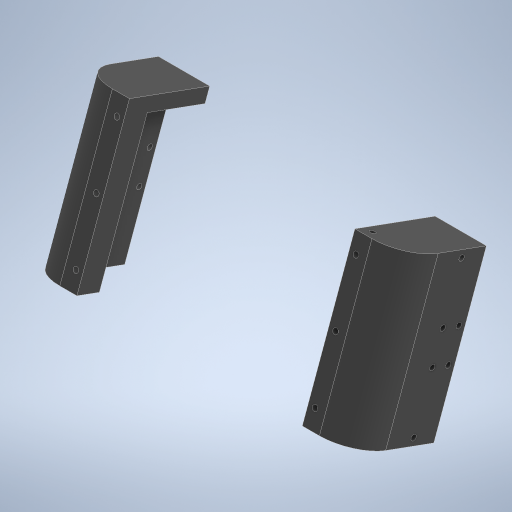
# Autodesk Inventor part: chest_cover_side
Saved by Autodesk Inventor 2024.1 (Build 281209000, 209)
## iProperties
Created: 2024-02-14
Part Number: chest_cover_side
Material: 一般
Document SubType Name: Modeling
Designer: hibik
Density: 1 g/cm^3
Appearance: 既定
Author: hibik
Autodesk Inventor part; units mm, degrees
ref_plane "YZ Plane" through (0, 0, 0) normal (1, 0, 0) x (0, 1, 0)
ref_plane "XZ Plane" through (0, 0, 0) normal (0, 1, 0) x (-1, 0, 0)
ref_plane "XY Plane" through (0, 0, 0) normal (0, 0, 1) x (1, 0, 0)
sketch "スケッチ1" plane through (0, 0, 0) normal (1, 0, 0) x (0, 1, 0)
  line L0 (0, 0) -> (33, 0)
  line L1 (33, 0) -> (3.8603, 10.606)
  line L2 (3.8603, 10.606) -> (0, 0)
  line L3 (33, 0) -> (3.8603, 10.606)
  line L4 (3.8603, 10.606) -> (5.2283, 14.3648)
  line L5 (5.2283, 14.3648) -> (34.3681, 3.7588)
  line L6 (34.3681, 3.7588) -> (33, 0)
  line L7 (5.2283, 14.3648) -> (0, 12.011)
  line L8 (0, 12.011) -> (3.8603, 10.606)
  line L9 (0, 0) -> (0, 12.011)
  circle A0 centre (2, 10.7181) radius 0.8
  line L10 (34.3681, 3.7588) -> (42.9186, 27.2511)
  line L11 (42.9186, 27.2511) -> (8.15, 39.9058)
  line L12 (8.15, 39.9058) -> (-0.4005, 16.4135)
  line L13 (-0.4005, 16.4135) -> (34.3681, 3.7588)
  line L14 (-0.4005, 16.4135) -> (8.15, 39.9058)
  line L15 (8.15, 39.9058) -> (50.4361, 24.5149)
  line L16 (50.4361, 24.5149) -> (41.8856, 1.0226)
  line L17 (41.8856, 1.0226) -> (-0.4005, 16.4135)
  line L18 (8.15, 39.9058) -> (-1.9502, 12.1558)
  line L19 (-1.9502, 12.1558) -> (2, 10.7181)
  line L20 (42.5697, 2.902) -> (0.2835, 18.2929)
  point P0 (0.2835, 18.2929)
  point P1 (-0.4005, 16.4135)
  point P2 (35.0521, 5.6382)
  point P3 (42.9186, 27.2511)
  dimension "d0" = 33
  dimension "d1" = 20
  dimension "d2" = 4
  dimension "d3" = 1.6
  dimension "d4" = 2
  dimension "d5" = 2
  dimension "d6" = 25
  dimension "d7" = 37
  dimension "d8" = 45
  dimension "d10" = 2
  constraints: 42 end point, 7 parallel, 6 perpendicular, 3 collinear, 3 point on line, 1 centre point, 1 coincident, 1 horizontal, 1 vertical
  measures "d0" distance of L0.start L0.end
  measures "d1" angle of L0 L1
  measures "d2" distance of L1.end L4.end
  measures "d3" diameter of A0
  measures "d4" distance from line of L7 L19.end
  measures "d5" distance from line of L9 L19.end
  measures "d6" distance between parallel lines of L5 L11
  measures "d7" distance between parallel lines of L12 L10
  measures "d8" distance between parallel lines of L12 L16
  measures "d10" distance between parallel lines of L17 L20
extrude "押し出し1" add sketch "スケッチ1" along normal blind 15 contours L5 L13 L12 L20 L10 | L10 L20 L16 L17 | L20 L12 L11 L10 | L10 L15 L16 L20
sketch "スケッチ2" plane through (0, 3.4515, 41.6159) normal (0, 0.3420201, 0.9396926) x (1, 0, 0)
  line L0 (0, 50) -> (5.2556, 50)
  line L1 (0, 0) -> (0, 50)
  circle A0 centre (2, 45) radius 0.8
  circle A1 centre (2, 10) radius 0.8
  circle A2 centre (2, 27.5) radius 0.8
  line L2 (0, 50) -> (4, 50)
  line L3 (4, 50) -> (4, 5)
  line L4 (4, 5) -> (0, 5)
  line L5 (0, 5) -> (0, 50)
  line L6 (0, 50) -> (0, 5) projected
  dimension "d13" = 1.6
  dimension "d14" = 1.6
  dimension "d15" = 1.6
  dimension "d18" = 5
  dimension "d19" = 17.5
  dimension "d21" = 17.5
  dimension "d22" = 2
  dimension "d23" = 4
  dimension "d30" = 5
  constraints: 12 end point, 3 centre point, 2 horizontal, 2 parallel, 2 vertical alignment, 1 collinear, 1 perpendicular
  measures "d13" diameter of A0
  measures "d14" diameter of A1
  measures "d15" diameter of A2
  measures "d18" distance from line of L4 A1.centre
  measures "d19" distance of A2.centre A0.centre
  measures "d21" distance of A2.centre A1.centre
  measures "d22" distance from line of A0.centre L5
  measures "d23" distance between parallel lines of L6 L3
  measures "d30" distance from line of L0 A0.centre
extrude "押し出し2" cut sketch "スケッチ2" against normal through all contours A0 | A1 | A2
ref_plane "作業平面1" through (-33, 0, 0) normal (-1, 0, 0) x (0, 0, 1)
mirror "ミラー1" about plane through (-33, 0, 0) normal (-1, 0, 0)
sketch "スケッチ4" plane through (-81, 2.3356, 23.9311) normal (-1, 0, 0) x (0, 0.3420201, 0.9396926)
  circle A0 centre (-6, 18) radius 0.8 projected
  circle A1 centre (-1, 18) radius 0.8 projected
  circle A2 centre (-1, 2) radius 0.8 projected
  line L0 (-8, 45) -> (17, 45) projected
  line L1 (-8, 0) -> (-8, 45) projected
  line L2 (17, 0) -> (-8, 0) projected
  line L3 (-8, 22.5) -> (0, 22.5)
  circle A3 centre (-6, 27) radius 0.8
  circle A4 centre (-1, 27) radius 0.8
  circle A5 centre (-1, 43) radius 0.8
  line L4 (17, 45) -> (17, 0) projected
  point P0 (-23.2867, 5.9901)
  constraints: 3 centre point, 3 symmetric about line, 2 end point, 1 midpoint, 3 other
extrude "押し出し4" cut sketch "スケッチ4" against normal through all contours A0 | A1 | A2 | A3 | A4 | A5
sketch "スケッチ5" plane through (-81, 41.8856, 1.0226) normal (0, 0.9396926, -0.3420201) x (1, 0, 0)
  circle A0 centre (83.3679, -22) radius 0.8 projected
  circle A1 centre (86.5298, -11.2421) radius 0.8 projected
  circle A2 centre (90.5298, -11.2421) radius 0.8 projected
  circle A3 centre (12.6321, -22) radius 0.8 projected
  circle A4 centre (9.4702, -11.2421) radius 0.8 projected
  circle A5 centre (5.4702, -11.2421) radius 0.8 projected
  point P0 (81, 15.2867)
extrude "押し出し5" cut sketch "スケッチ5" against normal through all
fillet "フィレット1" radius 10 2 edges at (-81, 29.293, 32.2104) (15, 29.293, 32.2104)
sketch "スケッチ6" plane through (-81, 41.8856, 1.0226) normal (0, 0.9396926, -0.3420201) x (1, 0, 0)
  line L0 (81, 0) -> (96, 0) projected
  line L1 (90.5, 0) -> (5.5, 0)
  line L2 (5.5, 0) -> (5.5, -18)
  line L3 (5.5, -18) -> (90.5, -18)
  line L4 (90.5, -18) -> (90.5, 0)
  line L5 (81, -25) -> (81, 0) projected
  line L6 (15, -25) -> (0, -25) projected
  line L7 (81, -25) -> (15, -25) construction
  point P0 (81, 15.2867)
  point P1 (81, -22.6101)
  point P2 (11, -25)
  point P3 (48, -25)
  point P4 (48, -18)
  dimension "d40" = 18
  dimension "d41" = 85
  constraints: 10 end point, 2 horizontal, 2 midpoint, 2 parallel, 1 perpendicular, 1 point on line, 1 vertical alignment
  measures "d40" distance of L3.end L1.start
  measures "d41" distance of L2.end L3.end
extrude "押し出し6" cut sketch "スケッチ6" against normal through all
sketch "スケッチ7" plane through (0, 50.4361, 24.5149) normal (0, 0.9396926, -0.3420201) x (1, 0, 0)
  circle A0 centre (2.3679, 3) radius 0.8 projected
  line L0 (9.5, 25) -> (9.5, 14.5574) projected
  arc A1 (9.5, 12.9585) -> (9.5, 14.5574) centre (9.5298, 13.7579) ccw projected
  line L1 (9.5, 12.9585) -> (9.5, 7) projected
  line L2 (9.5, 7) -> (0, 7) projected
  line L3 (0, 7) -> (0, 0) projected
  line L4 (0, 0) -> (5, 0) projected
  arc A2 (5, 0) -> (15, 10) centre (5, 10) ccw projected
  line L5 (15, 25) -> (15, 10) projected
  line L6 (9.5, 25) -> (15, 25) projected
  line L7 (-75.5, 14.5574) -> (-75.5, 25) projected
  line L8 (-75.5, 25) -> (-81, 25) projected
  line L9 (-81, 25) -> (-81, 10) projected
  arc A3 (-81, 10) -> (-71, 0) centre (-71, 10) ccw projected
  line L10 (-66, 0) -> (-71, 0) projected
  line L11 (-66, 7) -> (-66, 0) projected
  line L12 (-66, 7) -> (-75.5, 7) projected
  line L13 (-75.5, 7) -> (-75.5, 12.9585) projected
  arc A4 (-75.5, 14.5574) -> (-75.5, 12.9585) centre (-75.5298, 13.7579) ccw projected
  circle A5 centre (-68.3679, 3) radius 0.8 projected
  line L14 (15, 0) -> (0, 0)
  line L15 (0, 0) -> (0, 25)
  line L16 (0, 25) -> (15, 25)
  line L17 (15, 25) -> (15, 0)
  line L18 (-66, 0) -> (-81, 0)
  line L19 (-81, 0) -> (-81, 25)
  line L20 (-81, 25) -> (-66, 25)
  line L21 (-66, 25) -> (-66, 0)
  line L22 (15, 25) -> (15, 10) projected
  point P0 (0, 40.2867)
  constraints: 16 end point, 6 collinear, 4 parallel, 2 horizontal, 2 perpendicular, 1 point on line
extrude "押し出し7" add sketch "スケッチ7" against normal blind 4 contours L0 A1 L1 L2 L15 L16 | A4 L13 L12 L11 L10 A3 L9 L8 L7 | L7 L20 L21 L12 L13 A4 | A5
equation "\"d5\" = d4"
equation "\"d19\" = d21"
